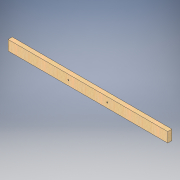
# Autodesk Inventor part: 56.25in 2x4
Saved by Autodesk Inventor 2017 (Build 210142000, 142)
## iProperties
Created: 2017-05-25
Part Number: 56.25in 2x4
Material: Pine, Radiata
Document SubType Name: Modeling
Designer: cas7
Density: 0.48 g/cm^3
Appearance: Pine - Coarse
Mass: 2322.87 g
Surface Area: 3696.77 cm^2
Volume: 4839.3 cm^3
Author: cas7
Autodesk Inventor part; units mm, degrees
ref_plane "YZ Plane" through (0, 0, 0) normal (1, 0, 0) x (0, 1, 0)
ref_plane "XZ Plane" through (0, 0, 0) normal (0, 1, 0) x (-1, 0, 0)
ref_plane "XY Plane" through (0, 0, 0) normal (0, 0, 1) x (1, 0, 0)
sketch "Sketch1" plane through (0, 0, 0) normal (0, 0, 1) x (1, 0, 0)
  line L0 (0, 0) -> (1428.75, 0)
  line L1 (1428.75, 0) -> (1428.75, 88.9)
  line L2 (1428.75, 88.9) -> (0, 88.9)
  line L3 (0, 88.9) -> (0, 0)
  dimension "d0" = 1428.75
  dimension "d1" = 88.9
  constraints: 8 end point, 2 parallel, 1 horizontal, 1 perpendicular
  measures "d0" distance of L2.end L1.end
  measures "d1" distance of L1.end L0.end
extrude "Extrusion1" add sketch "Sketch1" along normal blind 38.1
sketch "Sketch2" plane through (0, 0, 38.1) normal (0, 0, 1) x (1, 0, 0)
  line L0 (0, 88.9) -> (0, 0)
  line L1 (38.1, 88.9) -> (38.1, 0)
  line L2 (347.6625, 88.9) -> (347.6625, 0)
  line L3 (385.7625, 88.9) -> (385.7625, 0)
  line L4 (695.3377, 88.9) -> (695.3377, 0)
  line L5 (733.4377, 88.9) -> (733.4377, 0)
  line L6 (1043.0002, 88.9) -> (1043.0002, 0)
  line L7 (1081.1002, 88.9) -> (1081.1002, 0)
  line L8 (1390.6627, 88.9) -> (1390.6627, 0)
  line L9 (1428.7627, 88.9) -> (1428.7627, 0)
  line L10 (733.4377, 44.45) -> (888.2253, 44.45)
  line L11 (695.3377, 44.45) -> (540.5501, 44.45)
  dimension "d4" = 38.1
  dimension "d5" = 309.5625
  dimension "d6" = 38.1
  dimension "d7" = 309.5752
  dimension "d8" = 38.1
  dimension "d9" = 309.5625
  dimension "d10" = 38.1
  dimension "d11" = 309.5625
  dimension "d12" = 38.1
  dimension "d63" = 154.7876
  dimension "d64" = 154.7876
  constraints: 24 end point, 9 parallel, 2 coincident, 2 horizontal, 2 midpoint
  measures "d4" distance between parallel lines of L0 L1
  measures "d5" distance between parallel lines of L1 L2
  measures "d6" distance between parallel lines of L2 L3
  measures "d7" distance between parallel lines of L3 L4
  measures "d8" distance between parallel lines of L4 L5
  measures "d9" distance between parallel lines of L5 L6
  measures "d10" distance between parallel lines of L6 L7
  measures "d11" distance between parallel lines of L7 L8
  measures "d12" distance between parallel lines of L8 L9
  measures "d63" distance of L10.start L10.end
  measures "d64" distance of L11.start L11.end
hole "Hole3" at (540.5501, 44.45, 38.1) at (888.2253, 44.45, 38.1) direction (0, 0, -1) diameter 10.5918 end through all thread size "1/2-13 UNC" class "2B" standard "ANSI Unified Screw Threads"
body "Solid1"
